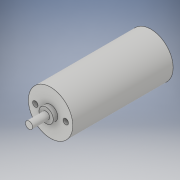
# Autodesk Inventor part: motor
Saved by Autodesk Inventor 2019 (Build 230136000, 136)
## iProperties
Created: 2020-03-05
Part Number: motor
Material: Generic
Document SubType Name: Modeling
Designer: Hugo Albarracin
Density: 1 g/cm^3
Appearance: Default
Author: Hugo Albarracin
Autodesk Inventor part; units mm, degrees
ref_plane "YZ Plane" through (0, 0, 0) normal (1, 0, 0) x (0, 1, 0)
ref_plane "XY Plane" through (0, 0, 0) normal (0, 0, 1) x (1, 0, 0)
sketch "Sketch1" plane through (0, 0, 0) normal (0, 0, 1) x (1, 0, 0)
  circle A0 centre (0, 0) radius 12.4
  dimension "d0" = 24.8
  constraints: 1 centre point, 1 coincident
  measures "d0" diameter of A0
extrude "Extrusion1" add sketch "Sketch1" against normal blind 56
sketch "Sketch2" plane through (0, 0, 0) normal (0, 0, 1) x (1, 0, 0)
  circle A0 centre (0, 0) radius 4
  dimension "d3" = 8
  constraints: 1 centre point, 1 coincident
  measures "d3" diameter of A0
extrude "Extrusion2" add sketch "Sketch2" along normal blind 2.5
sketch "Sketch3" plane through (0, 0, 2.5) normal (0, 0, 1) x (1, 0, 0)
  circle A0 centre (0, 0) radius 2
  dimension "d6" = 4
  constraints: 1 centre point, 1 coincident
  measures "d6" diameter of A0
extrude "Extrusion3" add sketch "Sketch3" along normal blind 9.5
sketch "Sketch4" plane through (0, 0, 0) normal (0, 0, 1) x (1, 0, 0)
  circle A0 centre (-8.5, 0) radius 1.5
  circle A1 centre (8.5, 0) radius 1.5
  circle A2 centre (0, 0) radius 2 projected
  line L0 (-8.5, 0) -> (0, 0) construction
  line L1 (0, 0) -> (8.5, 0) construction
  dimension "d9" = 3
  dimension "d10" = 3
  dimension "d11" = 17
  dimension "d12" = 8.5
  constraints: 4 end point, 2 centre point, 1 collinear, 1 horizontal
  measures "d9" diameter of A0
  measures "d10" diameter of A1
  measures "d11" distance of L1.end L0.start
  measures "d12" distance of L0.end L0.start
extrude "Extrusion4" cut sketch "Sketch4" against normal blind 8 contours A0 | A1
ref_plane "Work Plane1" through (0, -12.4, 0) normal (0, 1, 0) x (-1, 0, 0)
equation "\"d10\" = d9"
equation "\"d12\" = 0.5 * d11"
body "Solid1"
